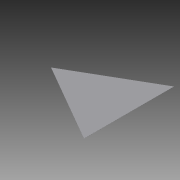
# Autodesk Inventor part: Triangle
Saved by Autodesk Inventor 2015 SP1 (Build 190203100, 203)
## iProperties
Created: 2016-02-24
Part Number: Triangle
Material: Generic
Document SubType Name: Modeling
Designer: jonesdm
Density: 1 g/cm^3
Appearance: Default
Author: jonesdm
Autodesk Inventor part; units mm, degrees
ref_plane "YZ Plane" through (0, 0, 0) normal (1, 0, 0) x (0, 1, 0)
ref_plane "XZ Plane" through (0, 0, 0) normal (0, 1, 0) x (-1, 0, 0)
ref_plane "XY Plane" through (0, 0, 0) normal (0, 0, 1) x (1, 0, 0)
sketch "Sketch1" plane through (0, 0, 0) normal (0, 1, 0) x (-1, 0, 0)
  line L0 (-659.9114, 762) -> (-659.9114, -762)
  line L1 (-659.9114, -762) -> (659.9114, 0)
  line L2 (-659.9114, 762) -> (659.9114, 0)
  point P0 (0, 0)
  point P1 (0, -381)
  dimension "d2" = 1524
  constraints: 6 end point, 2 equal length, 1 horizontal alignment, 1 midpoint, 1 vertical, 1 vertical alignment
  measures "d2" distance of L0.end L1.end
extrude "Extrusion1" add sketch "Sketch1" along normal blind 0.508
body "Solid1"
